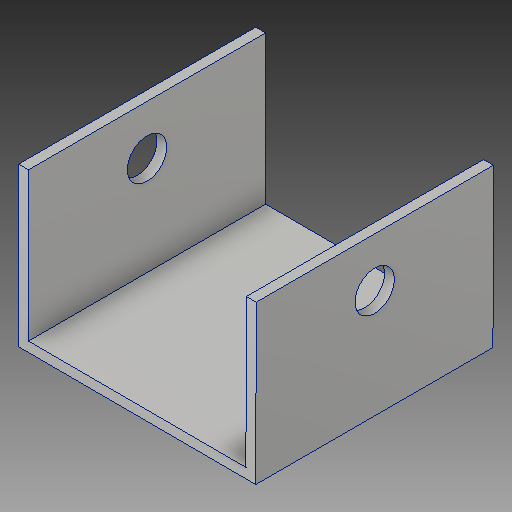
# Autodesk Inventor part: C Channel Connector
Saved by Autodesk Inventor 2017 (Build 210142000, 142)
## iProperties
Created: 2018-01-20
Part Number: C Channel Connector
Material: Aluminum 6061
Document SubType Name: Modeling
Designer: S346795925
Density: 2.7 g/cm^3
Appearance: Aluminum - Flat
Author: S346795925
Autodesk Inventor part; units mm, degrees
ref_plane "YZ Plane" through (0, 0, 0) normal (1, 0, 0) x (0, 1, 0)
ref_plane "XZ Plane" through (0, 0, 0) normal (0, 1, 0) x (-1, 0, 0)
ref_plane "XY Plane" through (0, 0, 0) normal (0, 0, 1) x (1, 0, 0)
sketch "Sketch1" plane through (0, 0, 0) normal (0, 0, 1) x (1, 0, 0)
  line L0 (0, 0) -> (76.1997, -0.2309)
  line L1 (76.1997, -0.2309) -> (76.3536, 50.5689)
  line L2 (0, 0) -> (0, 50.8)
  line L3 (0, 0) -> (50.8, 0) construction
  line L4 (3.175, 50.8) -> (3.175, 3.1654)
  line L5 (3.175, 3.1654) -> (73.0343, 2.9537)
  line L6 (73.0343, 2.9537) -> (73.1786, 50.5689)
  line L7 (0, 50.8) -> (3.175, 50.8)
  line L8 (73.1786, 50.5689) -> (76.3536, 50.5689)
  dimension "d0" = 76.2
  dimension "d1" = 50.8
  dimension "d2" = 90
  dimension "d3" = 50.8
  dimension "d4" = 90
  dimension "d5" = 3.175
  constraints: 18 end point, 4 perpendicular, 1 horizontal, 1 parallel, 1 vertical, 2 other
  measures "d0" distance of L0.start L0.end
  measures "d1" distance of L0.end L1.end
  measures "d2" angle of L1 L0
  measures "d3" distance of L0.start L2.end
  measures "d4" angle of L3 L2
  measures "d5" distance between parallel lines of L2 L4
extrude "Extrusion1" add sketch "Sketch1" along normal blind 76.2
sketch "Sketch3" plane through (76.3536, 50.5689, 76.2) normal (1, -0.003, 0) x (0, 0, -1)
  circle A0 centre (38.1, -15.875) radius 6.35
  line L0 (76.2, 0) -> (0, 0) projected
  line L1 (76.2, -50.8) -> (76.2, 0) projected
  line L2 (76.2, -50.8) -> (0, -50.8) projected
  point P0 (76.2, -47.625)
  dimension "d9" = 12.7
  dimension "d11" = 38.1
  dimension "d14" = 34.925
  constraints: 1 centre point
  measures "d9" diameter of A0
  measures "d11" distance from line of L1 A0.centre
  measures "d14" distance from line of L2 A0.centre
extrude "Extrusion2" cut sketch "Sketch3" against normal blind 103.1875
body "Solid1"
